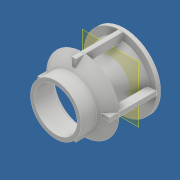
# Autodesk Inventor part: soundconev4
Saved by Autodesk Inventor 2017 (Build 210142000, 142)
## iProperties
Created: 2017-09-21
Part Number: soundconev4
Material: Generic
Document SubType Name: Modeling
Designer: Josh
Density: 1 g/cm^3
Appearance: Default
Author: Josh
Autodesk Inventor part; units mm, degrees
ref_plane "YZ Plane" through (0, 0, 0) normal (1, 0, 0) x (0, 1, 0)
ref_plane "XZ Plane" through (0, 0, 0) normal (0, 1, 0) x (-1, 0, 0)
ref_plane "XY Plane" through (0, 0, 0) normal (0, 0, 1) x (1, 0, 0)
sketch "Sketch1" plane through (0, 0, 0) normal (1, 0, 0) x (0, 1, 0)
  line L0 (0, -8.3) -> (7.6716, -8.3)
  line L1 (14, 0) -> (0, 0) construction
  line L2 (0, 0) -> (0, -8.3) construction
  line L3 (6.1716, -9.8) -> (0, -9.8)
  line L4 (0, -8.3) -> (0, -9.8)
  line L5 (25.1284, -11.1284) -> (25.1284, -14.1284)
  line L6 (25.1284, -14.1284) -> (26.6284, -14.1284)
  line L7 (14, 0) -> (22, 0)
  line L8 (25.1284, -11.1284) -> (14, 0)
  line L9 (26.6284, -14.1284) -> (26.6284, -11.1284)
  line L10 (26.6284, -11.1284) -> (22, 0)
  line L11 (7.6716, -8.3) -> (10.5, -11.1284)
  line L12 (10.5, -11.1284) -> (10.5, -14.1284)
  line L13 (10.5, -14.1284) -> (6.1716, -9.8)
  line L14 (25.1284, -11.1284) -> (10.5, -11.1284) construction
  dimension "d2" = 14
  dimension "d3" = 8.3
  dimension "d9" = 1.5
  dimension "d71" = 1.5
  dimension "d72" = 3
  dimension "d74" = 8
  dimension "d170" = 3
  dimension "d171" = 4
  dimension "d172" = 135
  dimension "d176" = 3.5
  constraints: 31 end point, 5 vertical, 3 horizontal, 3 parallel, 2 perpendicular
  measures "d2" distance of L1.start L1.end
  measures "d3" distance of L1.end L0.start
  measures "d9" distance between parallel lines of L0 L3
  measures "d71" distance of L5.end L6.end
  measures "d72" distance of L5.start L5.end
  measures "d74" distance of L1.start L7.end
  measures "d170" distance of L6.end L9.end
  measures "d171" distance of L11.end L0.end
  measures "d172" angle of L8 L1
  measures "d176" horizontal distance of L11.end L1.start
revolve "Revolution3" add sketch "Sketch1" angle 360 about axis through (0, 14, 0) along (0, -1, 0)
ref_plane "Work Plane2" through (0, 21.25, 0) normal (0, -1, 0) x (1, 0, 0)
sketch "Sketch13" plane through (0, 21.25, 0) normal (0, -1, 0) x (1, 0, 0)
  arc A0 (-13.9739, 0.8547) -> (-13.9739, -0.8547) centre (0, 0) ccw
  line L0 (0, 0) -> (-13.9739, -0.8547) construction
  line L1 (0, 0) -> (14, 0) construction
  line L2 (0, 0) -> (-13.9739, 0.8547) construction
  arc A1 (-10.4804, 0.641) -> (-10.4804, -0.641) centre (0, 0) ccw
  line L3 (0, 0) -> (-10.4804, 0.641) construction
  line L4 (0, 0) -> (-10.4804, -0.641) construction
  line L5 (-13.9739, -0.8547) -> (-10.4804, -0.641)
  line L6 (-13.9739, 0.8547) -> (-10.4804, 0.641)
  line L7 (0, 2.675) -> (0, -2.675)
  arc A2 (13.9739, -0.8547) -> (13.9739, 0.8547) centre (0, 0) ccw
  arc A3 (10.4804, -0.641) -> (10.4804, 0.641) centre (0, 0) ccw
  line L8 (13.9739, -0.8547) -> (10.4804, -0.641)
  line L9 (13.9739, 0.8547) -> (10.4804, 0.641)
  line L10 (-1.7678, 1.7678) -> (1.7678, -1.7678)
  line L11 (-1.7678, 1.7678) -> (3.2322, 1.7678) construction
  arc A4 (0.8547, 13.9739) -> (-0.8547, 13.9739) centre (0, 0) ccw
  arc A5 (0.641, 10.4804) -> (-0.641, 10.4804) centre (0, 0) ccw
  line L12 (0.8547, 13.9739) -> (0.641, 10.4804)
  line L13 (-0.8547, 13.9739) -> (-0.641, 10.4804)
  arc A6 (-0.8547, -13.9739) -> (0.8547, -13.9739) centre (0, 0) ccw
  arc A7 (-0.641, -10.4804) -> (0.641, -10.4804) centre (0, 0) ccw
  line L14 (-0.8547, -13.9739) -> (-0.641, -10.4804)
  line L15 (0.8547, -13.9739) -> (0.641, -10.4804)
  point P0 (0, 0)
  dimension "d150" = 14
  dimension "d151" = 176.5
  dimension "d152" = 7
  dimension "d153" = 10.5
  dimension "d154" = 7
  dimension "d155" = 5.35
  dimension "d156" = 5
  dimension "d157" = 45
  constraints: 32 end point, 16 point on circle, 12 symmetric about line, 8 centre point, 5 coincident, 2 equal length, 2 horizontal, 2 midpoint, 1 point on line, 1 vertical, 6 other
  measures "d150" radius of A0
  measures "d151" angle of L0 L1
  measures "d152" angle of L2 L0
  measures "d153" radius of A1
  measures "d154" angle of L3 L4
  measures "d155" distance of L7.start L7.end
  measures "d156" distance of L10.start L10.end
  measures "d157" angle of L10 L11
extrude "Extrusion7" add sketch "Sketch13" along normal blind 14.25 and the other way blind 4.75
body "Solid2"
